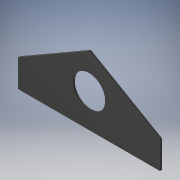
# Autodesk Inventor part: BA10
Saved by Autodesk Inventor 2017 (Build 210142000, 142)
## iProperties
Created: 2018-10-18
Part Number: BA10
Material: ABS Plastic
Document SubType Name: Modeling
Designer: Dell
Density: 1.06 g/cm^3
Appearance: Smooth - Black
Author: Dell
Autodesk Inventor part; units mm, degrees
ref_plane "YZ Plane" through (0, 0, 0) normal (1, 0, 0) x (0, 1, 0)
ref_plane "XZ Plane" through (0, 0, 0) normal (0, 1, 0) x (-1, 0, 0)
ref_plane "XY Plane" through (0, 0, 0) normal (0, 0, 1) x (1, 0, 0)
sketch "Sketch1" plane through (0, 0, 0) normal (0, 0, 1) x (1, 0, 0)
  line L0 (0, 0) -> (525.78, 0)
  line L1 (525.78, 0) -> (525.78, 101.6)
  line L2 (525.78, 101.6) -> (0, 101.6)
  line L3 (0, 101.6) -> (0, 0)
  line L4 (0, 101.6) -> (262.89, 253.3796)
  line L5 (262.89, 253.3796) -> (525.78, 101.6)
  point P0 (262.89, 101.6)
  dimension "d0" = 525.78
  dimension "d1" = 101.6
  dimension "d2" = 30
  constraints: 12 end point, 2 parallel, 1 horizontal, 1 midpoint, 1 perpendicular, 1 vertical alignment
  measures "d0" distance of L1.end L2.end
  measures "d1" distance of L0.end L1.end
  measures "d2" angle of L2 L5
extrude "Extrusion1" add sketch "Sketch1" along normal blind 6.35
sketch "Sketch7" plane through (0, 0, 6.35) normal (0, 0, 1) x (1, 0, 0)
  circle A0 centre (262.89, 123.3796) radius 60
  point P0 (0, 0)
  point P1 (262.89, 253.3796)
  dimension "d26" = 120
  dimension "d30" = 130
  constraints: 1 centre point, 1 vertical alignment
  measures "d26" diameter of A0
  measures "d30" distance of point (262.89, 253.38) A0.centre
extrude "Extrusion7" cut sketch "Sketch7" against normal through all
body "Solid1"
